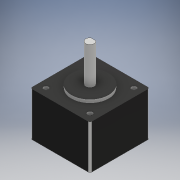
# Autodesk Inventor part: MotorNema14
Saved by Autodesk Inventor 2018.3 (Build 223284000, 284)
## iProperties
Created: 2018-06-16
Part Number: MotorNema14
Material: Типовые
Document SubType Name: Modeling
Designer: Leancher
Density: 1 g/cm^3
Appearance: По умолчанию
Author: Leancher
Autodesk Inventor part; units mm, degrees
ref_plane "YZ Plane" through (0, 0, 0) normal (1, 0, 0) x (0, 1, 0)
ref_plane "XZ Plane" through (0, 0, 0) normal (0, 1, 0) x (-1, 0, 0)
ref_plane "XY Plane" through (0, 0, 0) normal (0, 0, 1) x (1, 0, 0)
sketch "Эскиз1" plane through (0, 0, 0) normal (0, 0, 1) x (1, 0, 0)
  line L0 (-17.6, 17.6) -> (17.6, 17.6)
  line L1 (17.6, 17.6) -> (17.6, -17.6)
  line L2 (17.6, -17.6) -> (-17.6, -17.6)
  line L3 (-17.6, -17.6) -> (-17.6, 17.6)
  point P0 (13, -13)
  point P1 (-13, -13)
  point P2 (13, 13)
  point P3 (-13, 13)
  dimension "d0" = 35.2
  dimension "d1" = 35.2
  constraints: 8 end point, 2 parallel, 1 horizontal, 1 perpendicular
  measures "d0" distance of L1.end L2.end
  measures "d1" distance of L0.end L1.end
extrude "Выдавливание1" add sketch "Эскиз1" along normal blind 26
sketch "Эскиз2" plane through (0, 0, 26) normal (0, 0, 1) x (1, 0, 0)
  circle A0 centre (0, 0) radius 11
  dimension "d6" = 22
  constraints: 1 centre point, 1 coincident
  measures "d6" diameter of A0
extrude "Выдавливание2" add sketch "Эскиз2" along normal blind 2
sketch "Эскиз3" plane through (0, 0, 28) normal (0, 0, 1) x (1, 0, 0)
  circle A0 centre (0, 0) radius 11 projected
  circle A1 centre (0, 0) radius 2.5
  dimension "d9" = 5
  constraints: 1 centre point, 1 coincident
  measures "d9" diameter of A1
extrude "Выдавливание3" add sketch "Эскиз3" along normal blind 22 contours A1
sketch "Эскиз4" plane through (0, 0, 50) normal (0, 0, 1) x (1, 0, 0)
  line L0 (0, 2) -> (3.1194, 2)
  line L1 (3.1194, 2) -> (3.1194, 3.4913)
  line L2 (3.1194, 3.4913) -> (-4.7004, 3.4913)
  line L3 (-4.7004, 3.4913) -> (-4.7004, 2)
  line L4 (-4.7004, 2) -> (0, 2)
  constraints: 10 end point, 4 perpendicular, 1 point on line
extrude "Выдавливание4" cut sketch "Эскиз4" against normal blind 15
hole "Отверстие1" at (13, -13, 0) at (13, 13, 0) at (-13, 13, 0) at (-13, -13, 0) direction (0, 0, 1) diameter 3 end through all
fillet "Сопряжение1" radius 1 4 edges at (-17.6, -17.6, 13) (17.6, -17.6, 13) (17.6, 17.6, 13) (-17.6, 17.6, 13)
